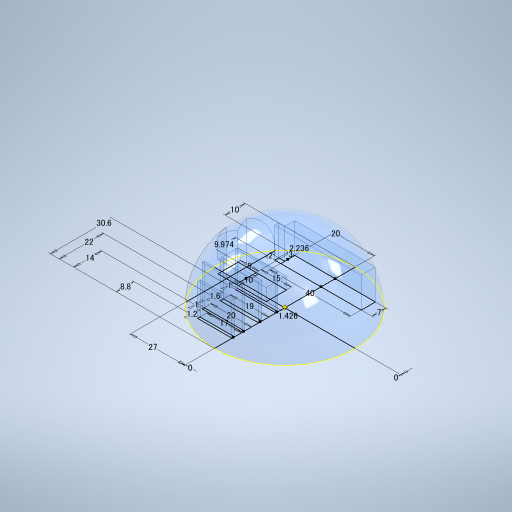
# Autodesk Inventor part: naibu
Saved by Autodesk Inventor 2023 (Build 270158000, 158)
## iProperties
Created: 2022-10-08
Part Number: naibu
Material: 一般
Document SubType Name: Modeling
Designer: ellie
Density: 1 g/cm^3
Appearance: 青 - 光沢
Author: ellie
Autodesk Inventor part; units mm, degrees
ref_plane "YZ Plane" through (0, 0, 0) normal (1, 0, 0) x (0, 1, 0)
ref_plane "XZ Plane" through (0, 0, 0) normal (0, 1, 0) x (-1, 0, 0)
ref_plane "XY Plane" through (0, 0, 0) normal (0, 0, 1) x (1, 0, 0)
sketch "スケッチ1" plane through (0, 0, 0) normal (0, 1, 0) x (-1, 0, 0)
  circle A0 centre (0, 0) radius 35
  line L0 (0, 0) -> (0, -35)
  line L1 (0, 0) -> (0, 35)
  dimension "d0" = 70
  constraints: 4 end point, 2 point on circle, 2 vertical, 1 centre point, 1 coincident
  measures "d0" diameter of A0
revolve "回転1" add sketch "スケッチ1" angle 180 about axis through (0, 0, 0) along (0, 0, 1) picked at (-2.5961, -23.0408) contours L1 L0 A0
sketch "スケッチ5" plane through (0, 0, 0) normal (0, -1, 0) x (1, 0, 0)
  line L0 (-20, -25) -> (20, -25)
  line L1 (20, -25) -> (20, -18)
  line L2 (20, -18) -> (-20, -18)
  line L3 (-20, -18) -> (-20, -25)
  line L4 (-20, -18) -> (-23, -18)
  line L5 (-23, -18) -> (-23, -20)
  line L6 (-23, -20) -> (-20, -20)
  line L7 (-20, -20) -> (-20, -18)
  line L8 (0, 26.2) -> (-17, 26.2)
  line L9 (-17, 26.2) -> (-17, 25)
  line L10 (-17, 25) -> (0, 25)
  line L11 (0, 25) -> (0, 26.2)
  line L12 (0, 21) -> (-20, 21)
  line L13 (-20, 21) -> (-20, 20)
  line L14 (-20, 20) -> (0, 20)
  line L15 (0, 20) -> (0, 21)
  line L16 (0, 13) -> (-19, 13)
  line L17 (-19, 13) -> (-19, 11.4)
  line L18 (-19, 11.4) -> (0, 11.4)
  line L19 (0, 11.4) -> (0, 13)
  line L20 (0, 4.4) -> (-20, 4.4)
  line L21 (-20, 4.4) -> (-20, 3.4)
  line L22 (-20, 3.4) -> (0, 3.4)
  line L23 (0, 3.4) -> (0, 4.4)
  circle A0 centre (0, 0) radius 35 projected
  circle A1 centre (0, 0) radius 35 projected
  line L24 (0, 35) -> (0, -35)
  line L25 (35, 0) -> (-35, 0)
  line L26 (-31.236, 1.9738) -> (-22.236, 1.9738)
  line L27 (-22.236, 1.9738) -> (-22.236, -8.0262)
  line L28 (-22.236, -8.0262) -> (-31.236, -8.0262)
  line L29 (-31.236, -8.0262) -> (-31.236, 1.9738)
  line L30 (-22.236, 1.9738) -> (-7.236, 1.9738)
  line L31 (-7.236, 1.9738) -> (-7.236, -8.0262)
  line L32 (-7.236, -8.0262) -> (-22.236, -8.0262)
  line L33 (-22.236, -8.0262) -> (-22.236, 1.9738)
  line L34 (-27, 22.2711) -> (-27, -22.2711)
  point P0 (0, -25)
  point P1 (0, -18)
  point P2 (-20, -20)
  point P3 (0, 25.6)
  point P4 (0, 20.5)
  point P5 (0, 12.2)
  point P6 (0, 3.9)
  point P7 (-22.236, -3.0262)
  point P8 (-20, -21.5)
  point P9 (-27, 1.9738)
  point P10 (-27, -8.0262)
  dimension "d12" = 40
  dimension "d13" = 7
  dimension "d21" = 3
  dimension "d22" = 2
  dimension "d23" = 17
  dimension "d24" = 1.2
  dimension "d27" = 20
  dimension "d28" = 1
  dimension "d30" = 19
  dimension "d31" = 1.6
  dimension "d33" = 1
  dimension "d88" = 0
  dimension "d89" = 0
  dimension "d90" = 10
  dimension "d92" = 20
  dimension "d93" = 8.8
  dimension "d94" = 14
  dimension "d95" = 22
  dimension "d96" = 30.6
  dimension "d97" = 9
  dimension "d98" = 10
  dimension "d99" = 1.4262
  dimension "d100" = 2.236
  dimension "d101" = 15
  dimension "d102" = 9.9738
  dimension "d113" = 27
  constraints: 70 end point, 16 parallel, 9 horizontal, 8 midpoint, 8 perpendicular, 6 point on circle, 4 point on line, 2 vertical
  measures "d12" distance of L2.end L1.end
  measures "d13" distance of L1.end L0.end
  measures "d21" distance of L6.end L5.end
  measures "d22" distance of L5.end L4.end
  measures "d23" distance of L10.end L9.end
  measures "d24" distance of L9.end L8.end
  measures "d27" distance of L14.end L13.end
  measures "d28" distance of L13.end L12.end
  measures "d30" distance of L18.end L17.end
  measures "d31" distance of L17.end L16.end
  measures "d33" distance of L21.end L20.end
  measures "d88" distance from line of L24 A0.centre
  measures "d89" distance from line of A1.centre L25
  measures "d90" distance from line of L0 L24.end
  measures "d92" distance between parallel lines of L3 L24
  measures "d93" distance from line of L8 L24.start
  measures "d94" distance from line of L12 L24.start
  measures "d95" distance from line of L16 L24.start
  measures "d96" distance from line of L20 L24.start
  measures "d97" distance of L27.end L28.end
  measures "d98" distance of L26.end L27.end
  measures "d99" distance between parallel lines of L26 L22
  measures "d100" horizontal distance of point (-22.236, -3.026) point (-20, -21.5)
  measures "d101" distance of L31.end L32.end
  measures "d102" distance between parallel lines of L32 L2
  measures "d113" distance between parallel lines of L34 L24
extrude "押し出し2" cut sketch "スケッチ5" against normal blind 15 contours L3 L2 L24 L0 | L24 L2 L1 L0 | L6 L5 L4 L3
extrude "押し出し12" cut sketch "スケッチ5" against normal blind 6 contours L31 L32 L27 L25 | L25 L27 L30 L31 | L34 L25 L27 L28 | L28 L29 L25 L34 | L25 L34 L26 L27 | L29 L26 L34 L25
extrude "押し出し13" cut sketch "スケッチ5" against normal blind 17.5 contours L22 L21 L20 L23
extrude "押し出し14" cut sketch "スケッチ5" against normal blind 17.5 contours L18 L17 L16 L19
extrude "押し出し15" cut sketch "スケッチ5" against normal blind 20 contours L15 L14 L13 L12
extrude "押し出し16" cut sketch "スケッチ5" against normal blind 16 contours L11 L10 L9 L8
extrude "押し出し17" cut sketch "スケッチ5" against normal blind 30 contours A0 L25 L29 L28 L34 | A0 L34 L26 L29 L25
